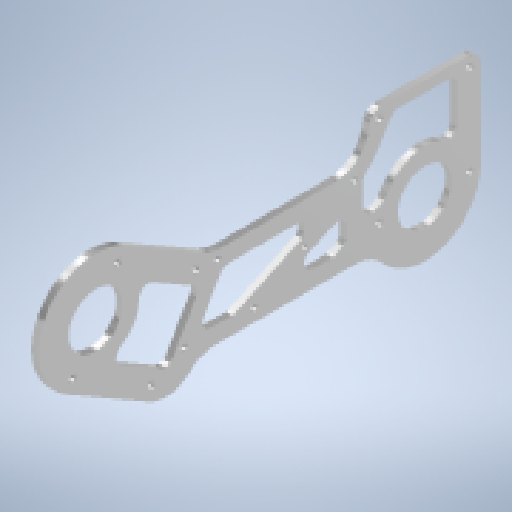
# Autodesk Inventor part: leg_under
Saved by Autodesk Inventor 2024.1 (Build 281209000, 209)
## iProperties
Created: 2023-08-04
Part Number: leg_under
Material: アルミニウム 6061
Document SubType Name: Modeling
Designer: hibik
Density: 2.7 g/cm^3
Appearance: アルミニウム - フラット
Author: hibik
Autodesk Inventor part; units mm, degrees
ref_plane "YZ Plane" through (0, 0, 0) normal (1, 0, 0) x (0, 1, 0)
ref_plane "XZ Plane" through (0, 0, 0) normal (0, 1, 0) x (-1, 0, 0)
ref_plane "XY Plane" through (0, 0, 0) normal (0, 0, 1) x (1, 0, 0)
sketch "スケッチ1" plane through (0, 0, 0) normal (1, 0, 0) x (0, 1, 0)
  line L0 (27, 0) -> (0, 0)
  line L1 (0, 0) -> (0, -65.8723)
  line L2 (0, -65.8723) -> (27, -65.8723)
  line L3 (27, -65.8723) -> (27, 0)
  line L4 (0, 0) -> (19.7037, 34.1277)
  line L5 (19.7037, 34.1277) -> (43.0863, 20.6277)
  line L6 (43.0863, 20.6277) -> (27, -7.2346)
  line L7 (27, 19.7654) -> (31.395, 27.3777)
  circle A0 centre (27, 19.7654) radius 6.25
  circle A1 centre (13.5, -57.0823) radius 6.25
  line L8 (13.5, -65.8723) -> (13.5, -57.0823)
  circle A2 centre (27, 19.7654) radius 13.5
  circle A3 centre (13.5, -57.0823) radius 13.5
  circle A4 centre (13.5, -57.0823) radius 13
  line L9 (37, -44.0823) -> (13.5, -44.0823)
  line L10 (13.5, -44.0823) -> (13.5, -70.0823)
  line L11 (13.5, -70.0823) -> (37, -70.0823)
  line L12 (37, -70.0823) -> (37, -44.0823)
  line L13 (8, 13.8564) -> (8, -44.7534)
  line L14 (8, -44.7534) -> (8, -45.303)
  point P0 (38.6913, 13.0154)
  point P1 (15.3087, 26.5154)
  point P2 (0, -57.0823)
  point P3 (27, -57.0823)
  point P4 (0, -57.0823)
  point P5 (27, -44.0823)
  point P6 (40.2685, 22.2546)
  point P7 (22.5215, 32.5009)
  point P8 (8, 0)
  point P9 (17.1401, -44.0823)
  point P10 (13.5, -44.0823)
  dimension "d23" = 26
  dimension "d0" = 27
  dimension "d4" = 150
  dimension "d5" = 90
  dimension "d6" = 27
  dimension "d12" = 8.79
  dimension "d13" = 8.79
  dimension "d14" = 12.5
  dimension "d17" = 100
  dimension "d24" = 23.5
  dimension "d30" = 8
  constraints: 30 end point, 6 coincident, 5 parallel, 4 centre point, 4 horizontal, 3 midpoint, 3 point on line, 3 vertical, 2 perpendicular, 2 point on circle, 2 tangent, 1 equal radius, 1 symmetric about line, 1 vertical alignment, 3 other
  measures "d0" distance of L1.end L2.end
  measures "d4" angle of L3 L6
  measures "d5" angle of L4 L5
  measures "d6" distance of L4.end L5.end
  measures "d12" distance from line of L7.start L5
  measures "d13" distance of L8.start point (13.5, -57.082)
  measures "d14" diameter of A0
  measures "d17" distance from line of L2 L4.end
  measures "d24" distance of L10.end L11.end
  measures "d30" distance between parallel lines of L13 L1
extrude "押し出し1" add sketch "スケッチ1" along normal blind 1.5 contours L3 L9 A3 L13 L0 | L0 L13 L4 A2 L6 L3 | L0 L4 L13 | A3 L9 A4 L14 | L9 L12 L11 A3 L2 L3 | L3 A3 L9 | A2 L5 | A3 L2 A4 L9 | A4 L10 A1 L8 L2 | L3 L2 A3 | A2 L5 | A4 L2 L8 A1 L10 | L2 L10 A4 | A3 L11 A4 L2 | L10 L8 A1 | A1 L8 L10 | L2 A4 L10 | A0 picked at (17.348, -69.6234)
extrude "押し出し2" cut sketch "スケッチ1" along normal blind 1.5 contours L10 L8 A1 | A1 L8 L10 | A0
fillet "フィレット1" radius 8 5 edges at (0.75, 27, -7.2346) (0.75, 27, -44.0823) (0.75, 8, -45.303) (0.75, 8, 0) (0.75, 0, 0)
fillet "フィレット2" radius 3 2 edges at (0.75, 37, -70.0823) (0.75, 37, -44.0823)
sketch "スケッチ6" plane through (1.5, 0, 0) normal (1, 0, 0) x (0, 0, -1)
  circle A0 centre (67.5823, 34.5) radius 0.85 projected
  circle A1 centre (46.5823, 34.5) radius 0.85 projected
  circle A2 centre (67.5823, 13.5) radius 0.85 projected
  circle A3 centre (46.5823, 13.5) radius 0.85 projected
  circle A4 centre (-6.8288, 7.4067) radius 0.85 projected
  circle A5 centre (-25.0154, 17.9067) radius 0.85 projected
  circle A6 centre (-14.5154, 36.0933) radius 0.85 projected
  circle A7 centre (3.6712, 25.5933) radius 0.85 projected
  line L0 (35.8933, 18.515) -> (30.098, 15.8126) projected
  line L1 (30.9432, 12) -> (35.3442, 12) projected
  line L2 (36.1894, 12.1874) -> (37.5838, 12.8376) projected
  line L3 (38.7385, 14.6502) -> (38.7385, 16.7024) projected
  line L4 (27.0251, 23) -> (11.2026, 23) projected
  line L5 (9.4706, 22) -> (5.4291, 15) projected
  line L6 (7.1612, 12) -> (12.0136, 12) projected
  line L7 (12.8588, 12.1874) -> (27.8704, 19.1874) projected
  line L8 (42.7385, 10.8278) -> (36.6744, 8) projected
  line L9 (3.1834, 8) -> (36.6744, 8) projected
  arc A8 (2.1834, 8.2679) -> (3.1834, 8) centre (3.1834, 10) ccw projected
  line L10 (-0.0294, 9.5455) -> (2.1834, 8.2679) projected
  arc A9 (-0.7615, 12.2776) -> (-0.0294, 9.5455) centre (0.9706, 11.2776) ccw projected
  line L11 (7.1612, 26) -> (-0.7615, 12.2776) projected
  arc A10 (8.8932, 27) -> (7.1612, 26) centre (8.8932, 25) ccw projected
  line L12 (40.7385, 27) -> (8.8932, 27) projected
  line L13 (42.7385, 10.8278) -> (42.7385, 25) projected
  circle A11 centre (-19.7654, 27) radius 6.25 projected
  circle A12 centre (57.0823, 13.5) radius 6.25 projected
  line L14 (-14.5154, 36.0933) -> (3.6712, 25.5933)
  line L15 (3.6712, 25.5933) -> (-6.8288, 7.4067)
  line L16 (-6.8288, 7.4067) -> (-25.0154, 17.9067)
  line L17 (-25.0154, 17.9067) -> (-14.5154, 36.0933)
  line L18 (5.3782, 28.0718) -> (-13.0154, 38.6913) projected
  line L19 (46.5823, 34.5) -> (67.5823, 34.5)
  line L20 (67.5823, 34.5) -> (67.5823, 13.5)
  line L21 (67.5823, 13.5) -> (46.5823, 13.5)
  line L22 (46.5823, 13.5) -> (46.5823, 34.5)
  line L23 (-16.0154, 33.4952) -> (4.6125, 21.5857)
  line L24 (4.6125, 21.5857) -> (-2.8875, 8.5953)
  line L25 (-2.8875, 8.5953) -> (-23.5154, 20.5048)
  line L26 (-23.5154, 20.5048) -> (-16.0154, 33.4952)
  line L27 (-2.8875, 8.5953) -> (3.1834, 8)
  circle A13 centre (-19.7654, 27) radius 10.25
  circle A14 centre (57.0823, 13.5) radius 10.25
  line L28 (49.5823, 34.5) -> (64.5823, 34.5)
  line L29 (64.5823, 34.5) -> (64.5823, 13.5)
  line L30 (64.5823, 13.5) -> (49.5823, 13.5)
  line L31 (49.5823, 13.5) -> (49.5823, 34.5)
  circle A15 centre (36.0823, 35) radius 12
  arc A16 (36.0823, 27) -> (44.0491, 34.2727) centre (36.0823, 35) ccw projected
  line L32 (38.7385, 13.376) -> (52.582, 19.8314)
  line L33 (46.5823, 29.1905) -> (49.5823, 34.5)
  arc A17 (35.3442, 12) -> (36.1894, 12.1874) centre (35.3442, 14) ccw projected
  arc A18 (37.5838, 12.8376) -> (38.7385, 14.6502) centre (36.7385, 14.6502) ccw projected
  arc A19 (27.8704, 19.1874) -> (27.0251, 23) centre (27.0251, 21) ccw projected
  arc A20 (11.2026, 23) -> (9.4706, 22) centre (11.2026, 21) ccw projected
  arc A21 (5.4291, 15) -> (7.1612, 12) centre (7.1612, 14) ccw projected
  arc A22 (12.0136, 12) -> (12.8588, 12.1874) centre (12.0136, 14) ccw projected
  arc A23 (30.098, 15.8126) -> (30.9432, 12) centre (30.9432, 14) ccw projected
  arc A24 (38.7385, 16.7024) -> (35.8933, 18.515) centre (36.7385, 16.7024) ccw projected
  circle A25 centre (8.8932, 25) radius 0.8 projected
  circle A26 centre (17.4111, 11) radius 0.8 projected
  circle A27 centre (28.9842, 17.5) radius 0.8 projected
  circle A28 centre (0.9706, 11.2776) radius 0.8 projected
  circle A29 centre (40.7385, 25) radius 0.8 projected
  arc A30 (42.7385, 25) -> (40.7385, 27) centre (40.7385, 25) ccw projected
  point P0 (0, 0)
  point P1 (8, 8)
  point P2 (-7.4164, 4.2819)
  point P3 (42.7385, 15.2413)
  point P4 (47.6605, 17.5364)
  point P5 (64.5823, 20.4866)
  point P6 (48.0718, 34.5)
  point P7 (42.7385, 25.0153)
  point P8 (-17.4648, 17.0115)
  point P9 (-0.7615, 12.2776)
  point P10 (-9.9648, 30.0019)
  point P11 (67.3323, 13.5)
  point P12 (42.7385, 25.0153)
  point P13 (27.138, 27)
  point P14 (46.5823, 17.0336)
  point P15 (46.8323, 13.5)
  point P16 (46.5823, 14.35)
  point P17 (47.4323, 13.5)
  point P18 (67.5823, 14.35)
  point P19 (66.7323, 13.5)
  point P20 (46.5823, 33.65)
  point P21 (47.4323, 34.5)
  point P22 (67.5823, 33.65)
  point P23 (66.7323, 34.5)
  dimension "d31" = 3
  dimension "d32" = 3
  dimension "d33" = 4
  dimension "d34" = 4
  dimension "d35" = 3
  dimension "d36" = 3
  dimension "d37" = 4
  constraints: 38 end point, 9 parallel, 5 coincident, 5 perpendicular, 5 point on line, 2 centre point, 2 horizontal, 1 collinear, 4 other
  measures "d31" distance from line of L23 L14.start
  measures "d32" distance from line of L25 A5.centre
  measures "d33" radial gap between concentric circles of A11 A13
  measures "d34" radial gap between concentric circles of A14 A12
  measures "d35" distance from line of L31 L19.start
  measures "d36" distance between parallel lines of L20 L29
extrude "押し出し6" cut sketch "スケッチ6" against normal through all contours A0 L20 L19 | L19 L20 A0 | L29 A14 L31 L19 | L20 L21 A14 A2 | A2 A14 L21 L20 | L31 A14 L32 L22 L33 | A14 L21 A2 | L22 L32 L13 A30 A15 | A2 L21 A14 | L19 L22 A1 | A1 L22 L19 | A14 L21 A3 | A3 L22 L21 A14 | A14 L21 L22 A3 | A3 L21 A14 | L11 L24 L25 L15 L23 | L15 L25 A13 L23 | L15 L14 A7 | A7 L14 L15 | L15 L16 A4 | A4 L16 L15 | A13 L17 L14 A6 | A6 L17 A13 | L14 L17 A13 A6 | A13 L17 A5 | A5 L16 L17 A13 | A6 A13 L17 | A5 A13 L17 L16 | L17 A13 A5 | A24 L3 A18 L2 A17 L1 A23 L0 | A19 L7 A22 L6 A21 L5 A20 L4 | A25 | A26 | A27 | A28 | A29
fillet "フィレット3" radius 2 10 edges at (0.75, 17.0115, 17.4648) (0.75, 30.0019, 9.9648) (0.75, 21.5857, -4.6125) (0.75, 8.5953, 2.8875) (0.75, 15.2413, -42.7385) (0.75, 17.5364, -47.6605) (0.75, 34.5, -49.5823) (0.75, 34.5, -64.5823) (0.75, 20.4866, -64.5823) (0.75, 25.0153, -42.7385)
